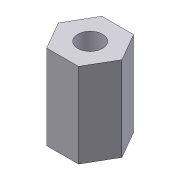
# Autodesk Inventor part: FOX-ME-117-05
Saved by Autodesk Inventor 2014 SP1 (Build 180222100, 222)
## iProperties
Created: 2012-08-02
Part Number: FOX-ME-117-05
Material: Aluminum-6061
Document SubType Name: Modeling
Designer: Robert Davis
Mass: 0.74252 g
Surface Area: 3.54207 cm^2
Volume: 0.273993 cm^3
Density: 2.71 g/cm^3
Description: AL THREADED SPACER
Appearance: Aluminum - Flat
Author: Robert Davis
Autodesk Inventor part; units mm, degrees
ref_plane "YZ Plane" through (0, 0, 0) normal (1, 0, 0) x (0, 1, 0)
ref_plane "XZ Plane" through (0, 0, 0) normal (0, 1, 0) x (-1, 0, 0)
ref_plane "XY Plane" through (0, 0, 0) normal (0, 0, 1) x (1, 0, 0)
sketch "Sketch1" plane through (0, 0, 0) normal (0, 0, 1) x (1, 0, 0)
  line L0 (1.8331, 3.175) -> (3.6662, 0)
  line L1 (3.6662, 0) -> (1.8331, -3.175)
  line L2 (1.8331, -3.175) -> (-1.8331, -3.175)
  line L3 (-1.8331, -3.175) -> (-3.6662, 0)
  line L4 (-3.6662, 0) -> (-1.8331, 3.175)
  line L5 (-1.8331, 3.175) -> (1.8331, 3.175)
  circle A0 centre (0, 0) radius 1.425
  dimension "d0" = 2.85
  dimension "d1" = 6.35
  constraints: 12 end point, 1 centre point, 13 other
  measures "d0" diameter of A0
  measures "d1" distance between parallel lines of L2 L5
extrude "Extrusion1" add sketch "Sketch1" along normal blind 9.75
body "Solid1"
